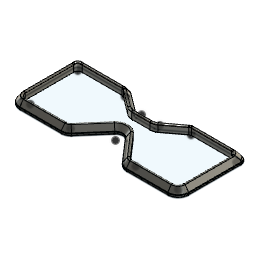
glasses v2 (Autodesk Fusion 360 design; units mm, degrees)
Autodesk Fusion 360 part; units mm, degrees
note: some values were not read from the file. Set by a fixed rule: which face or edge a step refers to.
sketch "Sketch1" plane through (0, 0, 0) normal (0, 0, 1) x (1, 0, 0)
  line L0 (0, 0) -> (0, 60) construction
  line L1 (0, 40) -> (-20, 40)
  line L2 (-20, 40) -> (-60, 70)
  line L3 (-60, 70) -> (-160, 70)
  line L4 (-160, 70) -> (-160, -60)
  line L5 (-160, -60) -> (-53.4549, -60)
  line L6 (-53.4549, -60) -> (-10, -10)
  line L7 (160, 70) -> (160, -60)
  line L8 (53.4549, -60) -> (10, -10)
  line L9 (160, -60) -> (53.4549, -60)
  line L10 (60, 70) -> (160, 70)
  line L11 (0, 40) -> (20, 40)
  line L12 (20, 40) -> (60, 70)
  arc A0 (10, -10) -> (-10, -10) centre (0, -18.691) ccw
  point P0 (0, 60)
  constraint coincident L0.start origin
  constraint vertical L0
  constraint coincident L0 L1.start
  constraint perpendicular L0 L1
  constraint perpendicular L0 L3
  constraint perpendicular L1 L4
  constraint perpendicular L4 L5
  constraint symmetric origin L0 L0.start
  constraint symmetric P0 L0 L0.end
  constraint symmetric L0 L1.start L11.start
  constraint symmetric L0 L1.end L11.end
  constraint symmetric L0 L2.end L10.start
  constraint symmetric L0 L3.end L7.start
  constraint symmetric L0 L4.end L7.end
  constraint symmetric L0 L5.end L8.start
  constraint symmetric L0 L6.end L8.end
  constraint tangent L6 A0
extrude "Extrude1" add sketch "Sketch1" along normal blind 5
fillet "Fillet1" radius 20 1 edges at (-160, -60, 2.5)
fillet "Fillet2" radius 18 2 edges at (-53.4549, -60, 2.5) (53.4549, -60, 2.5)
fillet "Fillet3" radius 20 1 edges at (160, -60, 2.5)
fillet "Fillet4" radius 10 2 edges at (-160, 70, 2.5) (160, 70, 2.5)
fillet "Fillet5" radius 8 4 edges at (-60, 70, 2.5) (60, 70, 2.5) (20, 40, 2.5) (-20, 40, 2.5)
sketch "Sketch2" plane through (0, 0, 5) normal (0, 0, 1) x (-1, 0, 0)
  arc A0 (-62.6667, -70) -> (-57.8667, -68.4) centre (-62.6667, -62) ccw
  line L0 (-57.8667, -68.4) -> (-22.1333, -41.6)
  arc A1 (-17.3333, -40) -> (-22.1333, -41.6) centre (-17.3333, -48) ccw
  line L1 (-17.3333, -40) -> (17.3333, -40)
  arc A2 (22.1333, -41.6) -> (17.3333, -40) centre (17.3333, -48) ccw
  line L2 (22.1333, -41.6) -> (57.8667, -68.4)
  arc A3 (57.8667, -68.4) -> (62.6667, -70) centre (62.6667, -62) ccw
  line L3 (62.6667, -70) -> (150, -70)
  arc A4 (150, -70) -> (160, -60) centre (150, -60) ccw
  line L4 (160, -60) -> (160, 40)
  arc A5 (160, 40) -> (140, 60) centre (140, 40) ccw
  line L5 (140, 60) -> (61.6592, 60)
  arc A6 (61.6592, 60) -> (48.0731, 53.8076) centre (61.6592, 42) ccw
  line L6 (48.0731, 53.8076) -> (10, 10)
  arc A7 (-10, 10) -> (10, 10) centre (0, 18.691) ccw
  line L7 (-10, 10) -> (-48.0731, 53.8076)
  arc A8 (-48.0731, 53.8076) -> (-61.6592, 60) centre (-61.6592, 42) ccw
  line L8 (-61.6592, 60) -> (-140, 60)
  arc A9 (-140, 60) -> (-160, 40) centre (-140, 40) ccw
  line L9 (-160, 40) -> (-160, -60)
  arc A10 (-160, -60) -> (-150, -70) centre (-150, -60) ccw
  line L10 (-150, -70) -> (-62.6667, -70)
extrude "Extrude2" add sketch "Sketch2" along normal blind 15 draft -35
sketch "Sketch3" plane through (0, 0, 0) normal (0, 0, -1) x (1, 0, 0)
  arc A0 (57.8667, -68.4) -> (62.6667, -70) centre (62.6667, -62) ccw
  line L0 (62.6667, -70) -> (150, -70)
  arc A1 (150, -70) -> (160, -60) centre (150, -60) ccw
  line L1 (160, -60) -> (160, 40)
  arc A2 (160, 40) -> (140, 60) centre (140, 40) ccw
  line L2 (140, 60) -> (61.6592, 60)
  arc A3 (61.6592, 60) -> (48.0731, 53.8076) centre (61.6592, 42) ccw
  line L3 (48.0731, 53.8076) -> (10, 10)
  arc A4 (-10, 10) -> (10, 10) centre (0, 18.691) ccw
  line L4 (-10, 10) -> (-48.0731, 53.8076)
  arc A5 (-48.0731, 53.8076) -> (-61.6592, 60) centre (-61.6592, 42) ccw
  line L5 (-61.6592, 60) -> (-140, 60)
  arc A6 (-140, 60) -> (-160, 40) centre (-140, 40) ccw
  line L6 (-160, 40) -> (-160, -60)
  arc A7 (-160, -60) -> (-150, -70) centre (-150, -60) ccw
  line L7 (-150, -70) -> (-62.6667, -70)
  arc A8 (-62.6667, -70) -> (-57.8667, -68.4) centre (-62.6667, -62) ccw
  line L8 (-57.8667, -68.4) -> (-22.1333, -41.6)
  arc A9 (-17.3333, -40) -> (-22.1333, -41.6) centre (-17.3333, -48) ccw
  line L9 (-17.3333, -40) -> (17.3333, -40)
  arc A10 (22.1333, -41.6) -> (17.3333, -40) centre (17.3333, -48) ccw
  line L10 (22.1333, -41.6) -> (57.8667, -68.4)
  arc A11 (-158, -60) -> (-150, -68) centre (-150, -60) ccw
  line L11 (-150, -68) -> (-62.6667, -68)
  arc A12 (-62.6667, -68) -> (-59.0667, -66.8) centre (-62.6667, -62) ccw
  line L12 (-59.0667, -66.8) -> (-23.3333, -40)
  arc A13 (-17.3333, -38) -> (-23.3333, -40) centre (-17.3333, -48) ccw
  line L13 (-17.3333, -38) -> (17.3333, -38)
  arc A14 (23.3333, -40) -> (17.3333, -38) centre (17.3333, -48) ccw
  line L14 (23.3333, -40) -> (59.0667, -66.8)
  arc A15 (59.0667, -66.8) -> (62.6667, -68) centre (62.6667, -62) ccw
  line L15 (62.6667, -68) -> (150, -68)
  arc A16 (150, -68) -> (158, -60) centre (150, -60) ccw
  line L16 (158, -60) -> (158, 40)
  arc A17 (158, 40) -> (140, 58) centre (140, 40) ccw
  line L17 (140, 58) -> (61.6592, 58)
  arc A18 (61.6592, 58) -> (49.5827, 52.4956) centre (61.6592, 42) ccw
  line L18 (49.5827, 52.4956) -> (11.5096, 8.688)
  arc A19 (-11.5096, 8.688) -> (11.5096, 8.688) centre (0, 18.691) ccw
  line L19 (-11.5096, 8.688) -> (-49.5827, 52.4956)
  arc A20 (-49.5827, 52.4956) -> (-61.6592, 58) centre (-61.6592, 42) ccw
  line L20 (-61.6592, 58) -> (-140, 58)
  arc A21 (-140, 58) -> (-158, 40) centre (-140, 40) ccw
  line L21 (-158, 40) -> (-158, -60)
  dimension "d10" = -2
fillet "Fillet6" radius 10 1 edges at (-149.7484, 59.7484, 19.6407)
fillet "Fillet7" radius 10 1 edges at (149.7484, 59.7484, 19.6407)
fillet "Fillet8" radius 8 2 edges at (-63.0839, 60.7484, 18.2126) (63.0839, 60.7484, 18.2126)
extrude "Extrude3" cut 1 faces at (92.2805, -10, 20) along direction (0, 0, -1) blind 10
extrude "Extrude4" cut 1 faces at (92.2805, -10, 10) along direction (0, 0, -1) blind 10
fillet "Fillet9" radius 2 22 edges at (-36.9641, -25.014, 20) (-58.5499, -48.8217, 20) (-100.8296, -49.4969, 20) (-146.7153, -46.7153, 20) (-149.4969, 5.6527, 20) (-147.2405, 57.2405, 20) (-103.4954, 59.4969, 20) (-63.6122, 59.1635, 20) (-45.0944, 45.6919, 20) (-23.1845, 30.4464, 20) (0, 29.4969, 20) (23.1845, 30.4464, 20) (45.0944, 45.6919, 20) (63.6122, 59.1635, 20) (103.4954, 59.4969, 20) (147.2405, 57.2405, 20) (149.4969, 5.6527, 20) (146.7153, -46.7153, 20) (100.8296, -49.4969, 20) (58.5499, -48.8217, 20) (36.9641, -25.014, 20) (0, 5.061, 20)
fillet "Fillet10" radius 2 22 edges at (54.1938, -58.3789, 0) (29.0366, -31.9038, 0) (0, -5.4421, 0) (-29.0366, -31.9038, 0) (-54.1938, -58.3789, 0) (-100.8296, -60, 0) (-154.1421, -54.1421, 0) (-160, 10, 0) (-157.0711, 67.0711, 0) (-106.3333, 70, 0) (-60.1368, 69.5895, 0) (-40, 55, 0) (-19.8632, 40.4105, 0) (0, 40, 0) (19.8632, 40.4105, 0) (40, 55, 0) (60.1368, 69.5895, 0) (106.3333, 70, 0) (157.0711, 67.0711, 0) (160, 10, 0) (154.1421, -54.1421, 0) (100.8296, -60, 0)
fillet "Fillet11" radius 2 22 edges at (-45.0944, 45.6919, 0) (-63.6122, 59.1635, 0) (-103.4954, 59.4969, 0) (-147.2405, 57.2405, 0) (-149.4969, 5.6527, 0) (-146.7153, -46.7153, 0) (-100.8296, -49.4969, 0) (-58.5499, -48.8217, 0) (-36.9641, -25.014, 0) (0, 5.061, 0) (36.9641, -25.014, 0) (58.5499, -48.8217, 0) (100.8296, -49.4969, 0) (146.7153, -46.7153, 0) (149.4969, 5.6527, 0) (147.2405, 57.2405, 0) (103.4954, 59.4969, 0) (63.6122, 59.1635, 0) (45.0944, 45.6919, 0) (23.1845, 30.4464, 0) (0, 29.4969, 0) (-23.1845, 30.4464, 0)
fillet "Fillet12" radius 2 159 faces at (59.5665, -52.8768, 14.8838) (87.7728, -52.6468, 15.2931) (146.5381, -51.3244, 14.8838) (151.0606, 20.8702, 15.6087) (149.4455, 52.4406, 13.9644) (152.8768, 53.1117, 15.1557) (157.7117, 23.7685, 8.268) (156.5046, -41.444, 9.902) (87.7728, -57.7117, 8.268) (60.313, -56.1222, 10.4466) (24.4182, -23.1015, 8.268) (42.4286, -33.0809, 15.4752) (43.3096, -32.3153, 5.8856) (42.3611, -33.1396, 0.1433) (56.9657, -50.1464, 0.0023) (87.7728, -49.4992, 1.9048) (149.2876, -46.6136, 0.0023) (151.1184, -9.5649, 0.0361) (150.1519, 54.1312, 0.2555) (116.0987, 59.8592, 0.852) (64.1663, 60.1341, 0.4049) (39.1898, 41.9957, 0.5858) (20.4741, 29.877, 1.3459) (5.7778, 29.5059, 1.8099) (-27.728, 32.8258, 1.3459) (-38.4554, 42.975, 0.0091) (-39.5413, 41.5271, 8.5523) (-27.7902, 32.735, 5.8856) (-5.7778, 29.4969, 5.8856) (22.8067, 30.3249, 9.7712) (39.5413, 41.5271, 8.5523) (65.0668, 59.4684, 7.3333) (65.2731, 59.4843, 11.2233) (116.0987, 59.4969, 7.3333) (149.4559, 52.2362, 4.6667) (149.471, 52.0478, 11.234) (149.4969, -9.5649, 8.5523) (149.4539, -40.9027, 5.8856) (113.8864, -49.4969, 5.8856) (58.2294, -48.6663, 5.8856) (145.1624, 62.0624, 16.1152) (148.3866, 63.8163, 13.3967) (117.9907, 67.7117, 8.268) (65.3008, 59.7206, 14.6197) (65.1873, 62.496, 15.4038) (116.0987, 60.1381, 15.1244) (143.1654, 60.485, 15.7664) (142.6924, 62.9334, 15.0749) (62.9358, 60.1858, 15.7452) (62.8209, 62.5667, 15.2591) (62.0868, 64.5226, 12.4519) (46.5235, 57.0323, 8.268) (38.7022, 42.646, 15.5642) (61.38, 59.3114, 15.4804) (60.1727, 61.2585, 15.0876) (18.9087, 29.684, 14.3376) (5.7778, 32.6468, 15.2931) (-21.2465, 30.0376, 14.3376) (-38.7022, 42.646, 15.5642) (-62.057, 58.4254, 13.9623) (-60.1501, 61.2132, 15.109) (-46.5235, 57.0323, 8.268) (-23.7283, 38.0667, 10.4466) (-5.7778, 37.7117, 8.268) (18.1773, 36.2164, 10.4466) (-62.1475, 69.2485, 6.0467) (-117.9907, 67.7117, 8.268) (-142.4406, 59.4455, 13.9644) (-143.1117, 62.8768, 15.1557) (-90.8921, 59.6886, 14.5114) (-90.8921, 59.4969, 7.3333) (-90.8921, 59.8592, 0.852) (-144.1312, 60.1519, 0.2555) (-149.785, 20.8702, 0.9659) (-144.2376, -50.585, 0.0023) (-113.8864, -49.5059, 1.8099) (-60.767, -51.3593, 0.0023) (-42.7332, -32.8162, 0.4279) (2.2434, 4.8443, 1.3459) (-155.8323, 23.7685, 0) (55.021, -58.6129, 1.3459) (23.6396, -23.7782, 0.1433) (10.4428, -7.71, 0.0023) (-9.1302, -9.0903, 3) (35.3821, -39.2051, 4) (53.4242, -58.0058, 4) (113.8864, -60, 3) (87.7728, -59.9909, 1.8099) (159.8675, -40.9464, 1.3459) (158.3785, -6.6667, 0.0361) (159.8788, 60.4706, 1.3459) (91.7778, 69.4475, 0.6198) (60.3109, 69.6075, 1.6215) (46.9285, 58.1695, 0.0361) (19.0247, 38.2406, 0.0023) (5.7778, 39.9977, 1.9048) (-20.6663, 38.6728, 0.0023) (-46.8726, 58.2439, 0.0564) (-62.3251, 69.9565, 1.6215) (-120.8889, 69.4475, 0.6198) (-159.6112, 62.3317, 1.3459) (-158.3785, 26.6667, 0.0361) (-159.8675, -40.9464, 1.3459) (-113.8864, -59.9909, 1.8099) (-53.4746, -57.908, 1.3459) (-35.9585, -38.7041, 0.4279) (-22.691, -24.6025, 3) (-49.2549, -55.0435, 4) (-87.7728, -60, 4) (-143.785, -59.6386, 3) (-160, -6.6667, 4) (-151.8925, 69.8193, 3) (-120.8889, 70, 4) (-58.1456, 68.6, 3) (-45.9556, 59.4667, 3) (-18.0189, 40.0294, 4) (-5.7778, 40, 4) (18.0189, 40.0294, 4) (34.0444, 50.5333, 4) (62.3236, 69.9926, 3) (91.7778, 70, 3) (159.9887, 60.4758, 4) (160, 26.6667, 3) (153.8016, -54.4747, 3) (-62.5865, 59.6075, 0.4049) (-62.2655, 58.5346, 7.3333) (-62.091, 58.4236, 11.2233) (-64.4286, 60.0103, 15.294) (-62.2032, 62.3608, 15.2591) (-61.6171, 64.366, 12.4519) (-65.2976, 59.5032, 13.9421) (-65.1122, 62.8714, 15.1192) (-16.3681, -1.4793, 9.7712) (-43.3096, -32.3153, 9.7712) (-60.9478, -49.4631, 9.7712) (-113.8864, -49.4969, 9.7712) (-140.9027, -49.4539, 5.8856) (-149.4969, -9.5649, 8.5523) (-142.2362, 59.4559, 4.6667) (-142.0478, 59.471, 11.234) (-152.0688, 55.1663, 16.1103) (-153.7465, 58.5549, 13.4233) (-157.7117, 23.7685, 8.268) (-149.3923, 52.8441, 14.0587) (-152.9334, 52.6924, 15.0749) (-150.7347, 20.8702, 15.5059) (-150.6516, -47.585, 14.8838) (-87.7728, -49.4993, 13.756) (-56.1297, -51.5973, 14.8838) (-28.7133, -19.3686, 15.5869) (-16.2858, -1.5659, 14.3376) (11.4955, -6.603, 9.902) (-38.8364, -36.203, 11.536) (-51.8831, -52.2799, 10.4466) (-113.8864, -57.7117, 8.268) (-141.444, -56.5046, 9.902) (-158.9326, 61.2121, 6.4075) (58.7329, 68.1103, 6.0467) (151.2121, 68.9326, 6.4075)
